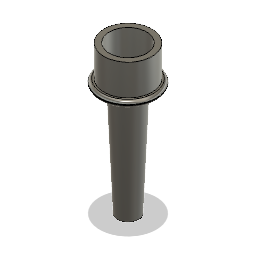
cap v9 (Autodesk Fusion 360 design; units mm, degrees)
Autodesk Fusion 360 part; units mm, degrees
note: some values were not read from the file. Set by a fixed rule: which sketch regions a step uses.
sketch "Sketch1" plane through (0, 0, 0) normal (0, 0, 1) x (1, 0, 0)
  line L0 (0, 0) -> (0, -36.322)
  line L1 (0, -36.322) -> (-2.286, -36.322)
  line L2 (-3.556, 0) -> (-2.286, -36.322)
  line L3 (-3.556, 0) -> (-3.556, 2.032)
  line L4 (0, 33.02) -> (0, -60.96) construction
  line L5 (-3.556, 2.032) -> (-5.7945, 2.032)
  line L6 (-6.096, 12.192) -> (0, 12.192)
  line L7 (0, 12.192) -> (0, 0)
  line L8 (-6.096, 12.192) -> (-5.7945, 2.032)
  dimension "d1" = 3.556
  dimension "d2" = 36.322
  dimension "d3" = 2.286
  dimension "d4" = 2.032
  dimension "d8" = 6.096
  dimension "d19" = 88.3
  measures "d1" distance of L0.start L2.start
  measures "d2" distance of L0.start L0.end
  measures "d3" distance of L0.end L1.end
  measures "d4" distance of L2.start L3.end
  measures "d8" distance of L6.start L6.end
  measures "d19" angle of L6 L8
sketch "Sketch2" plane through (0, 0, 0) normal (0, 0, 1) x (1, 0, 0)
  line L0 (-6.096, 12.192) -> (0, 12.192) construction
  line L1 (-6.096, 2.032) -> (-6.096, 12.192) construction
  line L2 (-3.556, 2.032) -> (-5.7945, 2.032) construction
  line L3 (-3.556, 0) -> (-3.556, 2.032) construction
  line L4 (-3.556, 0) -> (-2.286, -36.322) construction
  line L5 (0, -36.322) -> (-2.286, -36.322) construction
  line L6 (-7.874, 12.192) -> (-7.874, 2.032)
  line L7 (-9.3224, 0) -> (-9.3224, 2.032)
  line L8 (-7.874, 2.032) -> (-9.3224, 2.032)
  line L9 (-9.3224, 0) -> (-5.081, 0)
  line L10 (-7.874, 12.192) -> (0, 12.192)
  line L11 (0, 12.192) -> (0, -36.322)
  line L12 (0, -36.322) -> (-3.556, -36.322)
  line L13 (-3.556, -36.322) -> (-5.081, 0)
  dimension "d9" = 1.778
  dimension "d10" = 10.16
  dimension "d12" = 2.032
  dimension "d22" = 3.556
  measures "d9" distance of L0.start L6.start
  measures "d10" distance of L6.start L6.end
  measures "d12" distance of L7.start L7.end
  measures "d22" distance of L5.start L12.end
revolve "Revolve1" add sketch "Sketch2" angle 360 about axis through (0, 12.192, 0) along (0, -1, 0)
revolve "Revolve2" cut sketch "Sketch1" angle 360 about axis through (0, 12.192, 0) along (0, -1, 0)
fillet "Fillet1" radius 0.889 2 edges at (-8.6915, 2.032, 3.3711) (-8.6915, 0, 3.3711)
